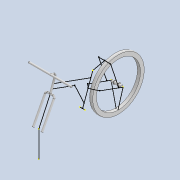
# Autodesk Inventor part: LW sketch
Saved by Autodesk Inventor 2021 (Build 250183000, 183)
## iProperties
Created: 2020-05-07
Part Number: LW sketch
Material: Generic
Document SubType Name: Modeling
Designer: Hannah
Appearance: Default
Surface Area: 5753.76 cm^2
Volume: 6332 cm^3
Author: Hannah
Autodesk Inventor part; units mm, degrees
ref_plane "Work Plane6" through (84.6427, 87.4734, -400.3058) normal (-1, 0, 0) x (0, 0.9396926, -0.3420201)
ref_plane "Work Plane5" through (-84.6427, 83.5886, -432.9589) normal (1, 0, 0) x (0, -0.9396926, 0.3420201)
ref_plane "Work Plane6" through (84.6427, 87.4734, -400.3058) normal (-1, 0, 0) x (0, 0.9396926, -0.3420201)
ref_plane "Work Plane3" through (-84.6427, 60, -486.347) normal (0, 1, 0) x (-1, 0, 0)
ref_plane "Work Plane1" through (-84.6427, 60, -486.347) normal (0, 0, 1) x (1, 0, 0)
ref_plane "Work Plane2" through (0, 0, 618) normal (0, 0, 1) x (1, 0, 0)
ref_plane "Work Plane4" through (-84.6427, -310, -486.347) normal (0, 1, 0) x (-1, 0, 0)
sketch3d "FEA outline"
sketch "Sketch4" plane through (0, 0, 0) normal (1, 0, 0) x (0, 1, 0)
  line L0 (1018.6374, 231.0623) -> (-500.8953, 784.127) projected
  line L1 (60, 633.1867) -> (42.899, 586.202)
  point P0 (0, 0)
  point P1 (60, -486.347)
  dimension "d64" = 50
  constraints: 2 end point, 1 perpendicular, 1 point on line, 1 vertical alignment
  measures "d64" distance of L1.start L1.end
ref_plane "Work Plane7" through (62.5, 60, 633.1867) normal (0, 0, 1) x (1, 0, 0)
sketch "Sketch2" plane through (62.5, 60, 633.1867) normal (0, 0, 1) x (1, 0, 0)
  line L0 (-84.5, -311) -> (-40.5, -311)
  line L1 (-40.5, -311) -> (-40.5, -363.4066)
  line L2 (-84.5, -363.4066) -> (-84.5, -311)
  line L3 (-125, 0) -> (0, 0) projected
  arc A0 (-84.5, -363.4066) -> (-40.5, -363.4066) centre (-62.5, -330) ccw
  line L4 (-12.5, -17.5) -> (-12.5, 0)
  line L5 (-12.5, 0) -> (-112.5, 0)
  line L6 (-112.5, 0) -> (-112.5, -17.5)
  line L7 (-94.5, -25) -> (-92.5, -25)
  line L8 (-92.5, -25) -> (-92.5, -17.5)
  line L9 (-94.5, -17.5) -> (-94.5, -25)
  line L10 (-32.5, -25) -> (-30.5, -25)
  line L11 (-30.5, -25) -> (-30.5, -17.5)
  line L12 (-32.5, -17.5) -> (-32.5, -25)
  line L13 (-112.5, -17.5) -> (-94.5, -17.5)
  line L14 (-92.5, -17.5) -> (-32.5, -17.5)
  line L15 (-30.5, -17.5) -> (-12.5, -17.5)
  point P0 (-62.5, -60)
  point P1 (-62.5, -311)
  point P2 (-62.5, -17.5)
  point P3 (-112.5, 0)
  point P4 (-62.5, -17.5)
  point P5 (-62.5, 0)
  dimension "TyreWidth" = 44
  dimension "d24" = 40
  dimension "BSD" = 622
  dimension "d26" = 660
  dimension "FrontHubSpacing" = 100
  dimension "d30" = 60
  dimension "d31" = 2
  dimension "d32" = 50
  dimension "d33" = 35
  constraints: 30 end point, 7 parallel, 6 horizontal, 6 perpendicular, 4 midpoint, 4 vertical alignment, 2 collinear, 2 equal length, 2 point on circle, 2 point on line, 1 centre point
  measures "TyreWidth" distance between parallel lines of L1 L2
  measures "d24" radius of A0
  measures "BSD" diameter of L0 L3
  measures "d26" diameter of A0.centre L3
  measures "FrontHubSpacing" distance of L6.end L4.start
  measures "d30" distance between parallel lines of L12 L8
  measures "d31" distance of L10.start L10.end
  measures "d32" diameter of L7 L3
  measures "d33" diameter of L13 L3
revolve "Revolution1" [suppressed]
ref_plane "Work Plane8" through (84.6427, 60, -486.347) normal (0, 0, 1) x (1, 0, 0)
sketch "Sketch3" plane through (84.6427, 255, -486.347) normal (0, 0, 1) x (1, 0, 0)
  line L0 (-106.6427, -506) -> (-62.6427, -506)
  line L1 (-62.6427, -506) -> (-62.6427, -558.4066)
  line L2 (-106.6427, -558.4066) -> (-106.6427, -506)
  line L3 (-37.8915, -195) -> (62.1085, -195)
  arc A0 (-106.6427, -558.4066) -> (-62.6427, -558.4066) centre (-84.6427, -525) ccw
  line L4 (-17.1427, -212.5) -> (-17.1427, -195)
  line L5 (-17.1427, -195) -> (-152.1427, -195)
  line L6 (-152.1427, -195) -> (-152.1427, -212.5)
  line L7 (-116.6427, -220) -> (-114.6427, -220)
  line L8 (-114.6427, -220) -> (-114.6427, -212.5)
  line L9 (-116.6427, -212.5) -> (-116.6427, -220)
  line L10 (-54.6427, -220) -> (-52.6427, -220)
  line L11 (-52.6427, -220) -> (-52.6427, -212.5)
  line L12 (-54.6427, -212.5) -> (-54.6427, -220)
  line L13 (-152.1427, -212.5) -> (-116.6427, -212.5)
  line L14 (-114.6427, -212.5) -> (-54.6427, -212.5)
  line L15 (-52.6427, -212.5) -> (-17.1427, -212.5)
  line L16 (-169.2853, -195) -> (0, -195) projected
  point P0 (-84.6427, -506)
  point P1 (-50, 0)
  point P2 (-84.6427, -212.5)
  point P3 (-84.6427, -195)
  point P4 (-84.6427, -255)
  dimension "d41" = 44
  dimension "d39" = 40
  dimension "d42" = 622
  dimension "d40" = 660
  dimension "RearHubWidth" = 135
  dimension "d35" = 60
  dimension "d36" = 2
  dimension "d37" = 50
  dimension "d34" = 35
  constraints: 32 end point, 7 parallel, 6 horizontal, 6 perpendicular, 3 collinear, 3 midpoint, 3 vertical alignment, 2 equal length, 2 point on circle, 2 point on line, 1 centre point
  measures "d41" distance between parallel lines of L1 L2
  measures "d39" radius of A0
  measures "d42" diameter of L0 L3
  measures "d40" diameter of A0.centre L3
  measures "RearHubWidth" distance of L6.end L4.start
  measures "d35" distance between parallel lines of L12 L8
  measures "d36" distance of L10.start L10.end
  measures "d37" diameter of L7 L3
  measures "d34" diameter of L13 L3
revolve "Revolution2" add sketch "Sketch3" angle 360 about axis through (46.7512, 60, -486.347) along (1, 0, 0) separate body
sketch "Sketch5" plane through (0, 0, 0) normal (1, 0, 0) x (0, 1, 0)
  circle A0 centre (640.537, 453.8138) radius 12.5
  circle A1 centre (406.3548, 453.9149) radius 12.5
  point P0 (0, 0)
  dimension "d67" = 25
  constraints: 2 centre point, 2 coincident, 1 equal radius
  measures "d67" diameter of A0
extrude "Extrusion1" add sketch "Sketch5" along normal mid plane 600 contours A0
sketch3d "placeholders"
  line L0 (62.5, 60, 633.1867) -> (62.5, 384.1526, 465.4067)
  arc A0 (62.5, 384.1526, 465.4067) -> (37.5, 406.3548, 453.9149) centre (37.5, 384.1526, 465.4067) ccw
  line L1 (37.5, 406.3548, 453.9149) -> (-37.5, 406.3548, 453.9149)
  arc A1 (-37.5, 406.3548, 453.9149) -> (-62.5, 384.1526, 465.4067) centre (-37.5, 384.1526, 465.4067) ccw
  line L2 (-62.5, 384.1526, 465.4067) -> (-62.5, 60, 633.1867)
  dimension "d6" = 125
  dimension "d8" = 80
  dimension "d15" = 600
  dimension "d17" = 25
  dimension "d18" = 25
  dimension "d65" = 390
  dimension "d66" = 80
  dimension "d76" = 25
sweep "Sweep1" add profiles "Sketch5" path "placeholders" contours A1
ref_plane "Work Plane9" through (0, 406.3548, 453.9149) normal (0, 0.9396926, -0.3420201) x (-1, 0, 0)
sketch "Sketch6" plane through (0, 406.3548, 453.9149) normal (0, 0.9396926, -0.3420201) x (-1, 0, 0)
  circle A0 centre (0, 0) radius 12.5
  point P0 (0, -565.522)
  point P1 (0, 0)
  dimension "d73" = 25
  constraints: 1 centre point, 1 coincident
  measures "d73" diameter of A0
sketch3d "placeholders for Sweep2"
  line L0 (0, 406.3548, 453.9149) -> (0, 589.6831, 387.1889)
  arc A0 (0, 589.6831, 387.1889) -> (0, 621.7259, 402.1307) centre (0, 598.2336, 410.6812) ccw
  line L1 (0, 621.7259, 402.1307) -> (0, 640.537, 453.8138)
  dimension "d6" = 125
  dimension "d8" = 80
  dimension "d15" = 600
  dimension "d17" = 25
  dimension "d18" = 25
  dimension "d65" = 390
  dimension "d66" = 80
  dimension "d76" = 25
sweep "Sweep2" add profiles "Sketch6" path "placeholders for Sweep2"
equation "\"d3\" = d2"
equation "\"d4\" = d2"
equation "\"d18\" = d17"
equation "\"d26\" = tyreOD - 2 * d24"
equation "\"d41\" = TyreWidth"
equation "\"d42\" = BSD"
equation "\"d40\" = tyreOD - 2 * d39"
equation "\"d2\" = 60"
equation "\"tyreOD\" = 740"
body "Solid1"
